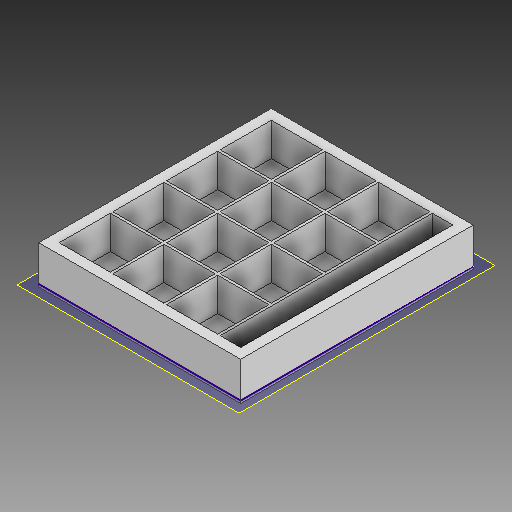
# Autodesk Inventor part: ключница
Saved by Autodesk Inventor 2026 (Build 300175000, 175)
## iProperties
Created: 2025-10-17
Part Number: ключница
Material: Типовые
Document SubType Name: Modeling
Designer: Admin
Density: 1 g/cm^3
Appearance: По умолчанию
Author: Admin
Autodesk Inventor part; units mm, degrees
ref_plane "YZ Plane" through (0, 0, 0) normal (1, 0, 0) x (0, 1, 0)
ref_plane "XZ Plane" through (0, 0, 0) normal (0, 1, 0) x (-1, 0, 0)
ref_plane "XY Plane" through (0, 0, 0) normal (0, 0, 1) x (1, 0, 0)
sketch "Эскиз1" plane through (0, 0, 0) normal (0, 1, 0) x (-1, 0, 0)
  line L0 (167.5, -227.5) -> (-167.5, -227.5)
  line L1 (-167.5, -227.5) -> (-167.5, 227.5)
  line L2 (-167.5, 227.5) -> (167.5, 227.5)
  line L3 (167.5, 227.5) -> (167.5, -227.5)
  line L4 (167.5, -227.5) -> (-167.5, 227.5) construction
  line L5 (-167.5, -227.5) -> (167.5, 227.5) construction
  point P0 (0, 0)
  dimension "d0" = 335
  dimension "d1" = 455
  constraints: 12 end point, 2 midpoint, 2 parallel, 1 horizontal, 1 perpendicular
  measures "d0" distance of L1.end L2.end
  measures "d1" distance of L0.end L1.end
extrude "Выдавливание1" add sketch "Эскиз1" along normal blind 70
sketch "Эскиз2" plane through (0, 70, 0) normal (0, 1, 0) x (1, 0, 0)
  line L0 (167.5, 227.5) -> (-167.5, 227.5) projected
  line L1 (-147.5, 227.5) -> (-147.5, -225.4146) construction
  line L2 (-167.5, 227.5) -> (-167.5, -227.5) projected
  line L3 (-167.5, 207.5) -> (167.5, 207.5)
  line L4 (-167.5, -207.5) -> (167.5, -207.5)
  line L5 (167.5, -227.5) -> (167.5, 227.5) projected
  line L6 (-167.5, -227.5) -> (167.5, -227.5) projected
  line L7 (162.5, 227.5) -> (162.5, -227.5)
  line L8 (-147.5, 207.5) -> (-47.5, 207.5)
  line L9 (-47.5, 207.5) -> (-47.5, 107.5)
  line L10 (-47.5, 107.5) -> (-147.5, 107.5)
  line L11 (-147.5, 107.5) -> (-147.5, 207.5)
  line L12 (-42.5, 107.5) -> (-42.5, 207.5)
  line L13 (-42.5, 207.5) -> (57.5, 207.5)
  line L14 (57.5, 207.5) -> (57.5, 107.5)
  line L15 (57.5, 107.5) -> (-42.5, 107.5)
  line L16 (62.5, 107.5) -> (62.5, 207.5)
  line L17 (62.5, 207.5) -> (162.5, 207.5)
  line L18 (162.5, 207.5) -> (162.5, 107.5)
  line L19 (162.5, 107.5) -> (62.5, 107.5)
  line L20 (-147.5, 2.5) -> (-147.5, 102.5)
  line L21 (-147.5, 102.5) -> (-47.5, 102.5)
  line L22 (-47.5, 102.5) -> (-47.5, 2.5)
  line L23 (-47.5, 2.5) -> (-147.5, 2.5)
  line L24 (-42.5, 2.5) -> (-42.5, 102.5)
  line L25 (-42.5, 102.5) -> (57.5, 102.5)
  line L26 (57.5, 102.5) -> (57.5, 2.5)
  line L27 (57.5, 2.5) -> (-42.5, 2.5)
  line L28 (62.5, 2.5) -> (62.5, 102.5)
  line L29 (62.5, 102.5) -> (162.5, 102.5)
  line L30 (162.5, 102.5) -> (162.5, 2.5)
  line L31 (162.5, 2.5) -> (62.5, 2.5)
  line L32 (-147.5, -102.5) -> (-147.5, -2.5)
  line L33 (-147.5, -2.5) -> (-47.5, -2.5)
  line L34 (-47.5, -2.5) -> (-47.5, -102.5)
  line L35 (-47.5, -102.5) -> (-147.5, -102.5)
  line L36 (-42.5, -102.5) -> (-42.5, -2.5)
  line L37 (-42.5, -2.5) -> (57.5, -2.5)
  line L38 (57.5, -2.5) -> (57.5, -102.5)
  line L39 (57.5, -102.5) -> (-42.5, -102.5)
  line L40 (62.5, -102.5) -> (62.5, -2.5)
  line L41 (62.5, -2.5) -> (162.5, -2.5)
  line L42 (162.5, -2.5) -> (162.5, -102.5)
  line L43 (162.5, -102.5) -> (62.5, -102.5)
  line L44 (-147.5, -207.5) -> (-147.5, -107.5)
  line L45 (-147.5, -107.5) -> (-47.5, -107.5)
  line L46 (-47.5, -107.5) -> (-47.5, -207.5)
  line L47 (-47.5, -207.5) -> (-147.5, -207.5)
  line L48 (-42.5, -207.5) -> (-42.5, -107.5)
  line L49 (-42.5, -107.5) -> (57.5, -107.5)
  line L50 (57.5, -107.5) -> (57.5, -207.5)
  line L51 (57.5, -207.5) -> (-42.5, -207.5)
  line L52 (62.5, -207.5) -> (62.5, -107.5)
  line L53 (62.5, -107.5) -> (162.5, -107.5)
  line L54 (162.5, -107.5) -> (162.5, -207.5)
  line L55 (162.5, -207.5) -> (62.5, -207.5)
  point P0 (0, 0)
  point P1 (162.5, -207.5)
  point P2 (162.5, 207.5)
  dimension "d4" = 20
  dimension "d5" = 20
  dimension "d6" = 20
  dimension "d7" = 5
  dimension "d8" = 100
  dimension "d9" = 100
  dimension "d12" = 105
  dimension "d15" = 105
  constraints: 104 end point, 8 point on line, 4 horizontal, 2 parallel, 2 perpendicular, 2 vertical, 88 other
  measures "d4" distance between parallel lines of L2 L1
  measures "d5" distance between parallel lines of L3 L0
  measures "d6" distance between parallel lines of L6 L4
  measures "d7" distance between parallel lines of L5 L7
  measures "d8" distance of L9.end L10.end
  measures "d9" distance of L8.end L9.end
  measures "d12" distance of L10.end L12.start
  measures "d15" distance of L10.end L20.start
extrude "Выдавливание2" cut sketch "Эскиз2" against normal blind 65 contours L7 L19 L16 L3 | L4 L52 L53 L7 | L3 L9 L10 L11 | L14 L15 L12 L3 | L7 L31 L28 L29 | L44 L45 L46 L4 | L4 L48 L49 L50 | L43 L40 L41 L7 | L20 L21 L22 L23 | L24 L25 L26 L27 | L32 L33 L34 L35 | L36 L37 L38 L39
sketch "Эскиз6" plane through (0, 0, 0) normal (0, -1, 0) x (1, 0, 0)
  line L0 (167.5, -227.5) -> (227.5, -227.5)
  line L1 (227.5, -227.5) -> (227.5, 227.5)
  line L2 (227.5, 227.5) -> (167.5, 227.5)
  line L3 (167.5, 227.5) -> (167.5, -227.5)
  point P0 (0, 0)
  dimension "d29" = 60
  constraints: 8 end point, 2 parallel, 1 horizontal, 1 perpendicular
  measures "d29" distance of L2.end L1.end
extrude "Выдавливание5" add sketch "Эскиз6" against normal blind 70
sketch "Эскиз7" plane through (0, 70, 0) normal (0, 1, 0) x (1, 0, 0)
  line L0 (227.5, 227.5) -> (-167.5, 227.5) projected
  line L1 (207.5, 227.5) -> (207.5, -226.0922)
  line L2 (227.5, -227.5) -> (227.5, 227.5) projected
  line L3 (227.5, 207.5) -> (-167.5, 207.5)
  line L4 (207.5, 207.5) -> (167.5, 207.5)
  line L5 (167.5, 207.5) -> (167.5, -207.5)
  line L6 (167.5, -207.5) -> (207.5, -207.5)
  line L7 (207.5, -207.5) -> (207.5, 207.5)
  point P0 (0, 0)
  dimension "d32" = 20
  dimension "d33" = 20
  dimension "d34" = 40
  dimension "d35" = 415
  constraints: 12 end point, 4 point on line, 3 perpendicular, 2 parallel, 1 horizontal
  measures "d32" distance between parallel lines of L2 L1
  measures "d33" distance between parallel lines of L3 L0
  measures "d34" distance of L5.end L6.end
  measures "d35" distance of L4.end L5.end
extrude "Выдавливание6" cut sketch "Эскиз7" against normal blind 65 contours L1 L6 L5 L3
ref_plane "РабПлоскость2" through (0, 0, 0) normal (0, -1, 0) x (1, 0, 0)
sketch "Эскиз8" plane through (0, 0, 0) normal (0, -1, 0) x (1, 0, 0)
  point P0 (0, 0)
sketch "Эскиз9" plane through (0, 0, 0) normal (0, -1, 0) x (1, 0, 0)
  line L0 (-167.5, -227.5) -> (-167.5, 227.5) projected
  line L1 (227.5, -227.5) -> (-167.5, -227.5) projected
  line L2 (-167.5, 227.5) -> (227.5, 227.5)
  line L3 (227.5, 227.5) -> (227.5, -227.5)
  line L4 (227.5, -227.5) -> (-167.5, -227.5)
  line L5 (-167.5, -227.5) -> (-167.5, 227.5)
  point P0 (0, 0)
  constraints: 8 end point, 2 parallel, 1 horizontal, 1 perpendicular
sketch "Эскиз10" plane through (0, 0, 0) normal (0, -1, 0) x (1, 0, 0)
  point P0 (0, 0)
sketch "Эскиз11" plane through (0, 0, 0) normal (0, -1, 0) x (1, 0, 0)
  line L0 (-167.5, -227.5) -> (-167.5, 227.5) projected
  line L1 (227.5, -227.5) -> (-167.5, -227.5) projected
  line L2 (-167.5, 227.5) -> (227.5, 227.5)
  line L3 (227.5, 227.5) -> (227.5, -227.5)
  line L4 (227.5, -227.5) -> (-167.5, -227.5)
  line L5 (-167.5, -227.5) -> (-167.5, 227.5)
  point P0 (0, 0)
  constraints: 8 end point, 2 parallel, 1 horizontal, 1 perpendicular
extrude "Выдавливание7" add sketch "Эскиз11" along normal blind 5
sketch "Эскиз12" plane through (0, -5, 0) normal (0, -1, 0) x (1, 0, 0)
  line L0 (-147.5, -229.7416) -> (-147.5, 227.5)
  line L1 (-167.5, 227.5) -> (227.5, 227.5) projected
  line L2 (-167.5, 227.5) -> (-167.5, -227.5) projected
  line L3 (-167.5, -207.5) -> (227.5, -207.5)
  line L4 (227.5, 227.5) -> (227.5, -227.5) projected
  line L5 (-167.5, -227.5) -> (227.5, -227.5) projected
  line L6 (207.5, 207.5) -> (167.5, 207.5) projected
  line L7 (-147.5, -207.5) -> (207.5, -207.5)
  line L8 (207.5, -207.5) -> (207.5, 207.5)
  line L9 (207.5, 207.5) -> (-147.5, 207.5)
  line L10 (-147.5, 207.5) -> (-147.5, -207.5)
  point P0 (0, 0)
  dimension "d41" = 20
  dimension "d42" = 20
  constraints: 12 end point, 5 point on line, 2 horizontal, 2 parallel, 1 perpendicular, 1 vertical
  measures "d41" distance between parallel lines of L2 L0
  measures "d42" distance between parallel lines of L5 L3
extrude "Выдавливание8" cut sketch "Эскиз12" against normal blind 5 contours L0 L9 L6 L8 L3
